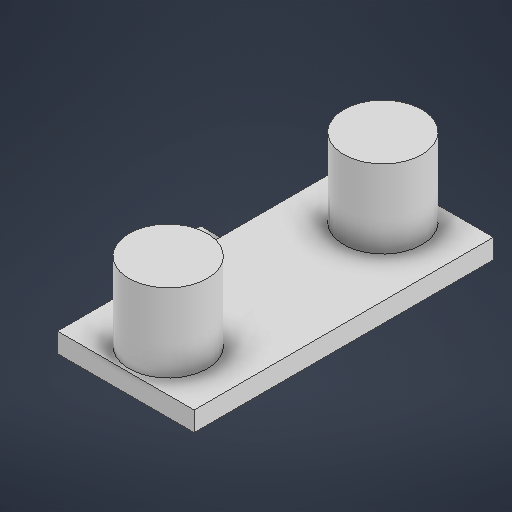
# Autodesk Inventor part: Sensore ultrasuoni
Saved by Autodesk Inventor 2026.2 (Build 302298000, 298)
## iProperties
Created: 2026-01-19
Part Number: Sensore ultrasuoni
Material: Generic
Document SubType Name: Modeling
Designer: ASUS
Density: 1 g/cm^3
Appearance: Default
Author: ASUS
Autodesk Inventor part; units mm, degrees
ref_plane "YZ Plane" through (0, 0, 0) normal (1, 0, 0) x (0, 1, 0)
ref_plane "XZ Plane" through (0, 0, 0) normal (0, 1, 0) x (-1, 0, 0)
ref_plane "XY Plane" through (0, 0, 0) normal (0, 0, 1) x (1, 0, 0)
sketch "Sketch1" plane through (0, 0, 0) normal (0, 1, 0) x (-1, 0, 0)
  line L0 (0, 0) -> (-21, 0)
  line L1 (-21, 0) -> (-21, 46)
  line L2 (-21, 46) -> (0, 46)
  line L3 (0, 46) -> (0, 0)
  dimension "d0" = 21
  dimension "d1" = 46
  constraints: 8 end point, 2 parallel, 1 horizontal, 1 perpendicular
  measures "d0" distance of L1.end L2.end
  measures "d1" distance of L0.end L1.end
extrude "Extrusion1" add sketch "Sketch1" along normal blind 3
sketch "Sketch2" plane through (0, 3, 0) normal (0, 1, 0) x (1, 0, 0)
  line L0 (21, 0) -> (0, 0) projected
  line L1 (0, -46) -> (21, -46) projected
  circle A0 centre (10.5, -39.5) radius 6
  line L2 (0, 0) -> (0, -46) projected
  line L3 (0, -23) -> (21, -23)
  line L4 (21, -46) -> (21, 0) projected
  circle A1 centre (10.5, -6.5) radius 6
  dimension "d6" = 12
  constraints: 2 centre point, 2 end point, 2 midpoint, 1 symmetric about line, 1 other
  measures "d6" diameter of A0
extrude "Extrusion2" add sketch "Sketch2" along normal blind 12 contours A0 | A1
sketch "Sketch3" plane through (0, 0, 0) normal (-1, 0, 0) x (0, 0, 1)
  line L0 (46, 0) -> (0, 0) projected
  line L1 (18, 0) -> (28, 0)
  line L2 (28, 0) -> (28, -4.5)
  line L3 (28, -4.5) -> (18, -4.5)
  line L4 (18, -4.5) -> (18, 0)
  dimension "d11" = 10
  constraints: 8 end point, 2 parallel, 1 horizontal, 1 perpendicular, 1 point on line
  measures "d11" distance of L2.end L3.end
extrude "Extrusion3" add sketch "Sketch3" along normal blind 6
sketch "Sketch4" plane through (0, 0, 0) normal (1, 0, 0) x (0, 0, -1)
  line L0 (-28, -4.5) -> (-28, 0) projected
  line L1 (-18, 0) -> (-18, -4.5) projected
  line L2 (-28, 0) -> (-18, 0)
  line L3 (-18, 0) -> (-18, -4.5)
  line L4 (-18, -4.5) -> (-28, -4.5)
  line L5 (-28, -4.5) -> (-28, 0)
  point P0 (0, 0)
  constraints: 8 end point, 2 parallel, 1 horizontal, 1 perpendicular
extrude "Extrusion4" add sketch "Sketch4" along normal blind 2
body "Solid1"
